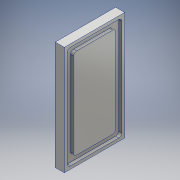
# Autodesk Inventor part: plateEnd
Saved by Autodesk Inventor 2016 (Build 200138000, 138)
## iProperties
Created: 2016-07-15
Part Number: plateEnd
Material: Aluminum 6061
Document SubType Name: Modeling
Designer: Jonathan
Density: 2.7 g/cm^3
Appearance: Aluminum - Flat
Author: Jonathan
Autodesk Inventor part; units mm, degrees
ref_plane "YZ Plane" through (0, 0, 0) normal (1, 0, 0) x (0, 1, 0)
ref_plane "XZ Plane" through (0, 0, 0) normal (0, 1, 0) x (-1, 0, 0)
ref_plane "XY Plane" through (0, 0, 0) normal (0, 0, 1) x (1, 0, 0)
sketch "Sketch1" plane through (0, 0, 0) normal (1, 0, 0) x (0, 1, 0)
  line L0 (31.75, 57.15) -> (-31.75, 57.15)
  line L1 (-31.75, 57.15) -> (-31.75, -57.15)
  line L2 (-31.75, -57.15) -> (31.75, -57.15)
  line L3 (31.75, -57.15) -> (31.75, 57.15)
  point P0 (0, 0)
  point P1 (31.75, 0)
  point P2 (0, 57.15)
  dimension "d0" = 114.3
  dimension "d1" = 63.5
  constraints: 8 end point, 2 midpoint, 2 parallel, 1 horizontal, 1 horizontal alignment, 1 perpendicular, 1 vertical alignment
  measures "d0" distance of L2.end L0.start
  measures "d1" distance of L1.end L2.end
extrude "Extrusion1" add sketch "Sketch1" along normal blind 9.525
sketch "Sketch3" plane through (9.525, 0, 0) normal (1, 0, 0) x (0, 0, -1)
  line L0 (-53.975, 28.575) -> (53.975, 28.575)
  line L1 (53.975, 28.575) -> (53.975, -28.575)
  line L2 (53.975, -28.575) -> (-53.975, -28.575)
  line L3 (-53.975, -28.575) -> (-53.975, 28.575)
  line L4 (-47.498, 22.098) -> (47.498, 22.098)
  line L5 (47.498, 22.098) -> (47.498, -22.098)
  line L6 (47.498, -22.098) -> (-47.498, -22.098)
  line L7 (-47.498, -22.098) -> (-47.498, 22.098)
  point P0 (0, 0)
  point P1 (0, 0)
  point P2 (-53.975, 0)
  point P3 (0, 28.575)
  dimension "d8" = 57.15
  dimension "d9" = 107.95
  dimension "d14" = 6.477
  constraints: 16 end point, 4 parallel, 2 midpoint, 2 perpendicular, 1 horizontal, 1 horizontal alignment, 1 vertical alignment, 3 other
  measures "d8" distance of L0.end L1.end
  measures "d9" distance of L0.start L0.end
  measures "d14" distance between parallel lines of L0 L4
extrude "Extrusion3" cut sketch "Sketch3" against normal blind 3.175
fillet "Fillet1" radius 3.175 8 edges at (7.9375, 28.575, 53.975) (7.9375, -28.575, 53.975) (7.9375, -28.575, -53.975) (7.9375, 28.575, -53.975) (7.9375, -22.098, -47.498) (7.9375, 22.098, -47.498) (7.9375, 22.098, 47.498) (7.9375, -22.098, 47.498)
body "Solid1"
